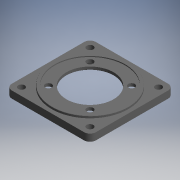
# Autodesk Inventor part: 2683767 EAMF-U-140A-120G-S1---(ADAX)
Saved by Autodesk Inventor 2017.3 (Build 213256000, 256)
## iProperties
Part Number: 2683767 EAMF-U-140A-120G-S1---(ADAX)
Material: Generic
Catalog Web Link: www.cadenas.de
Description: EAMF-U-E-xx-(ADAX)-adapter plate
Vendor: FESTO
Document SubType Name: Modeling
Designer: partserver
Manufacturer: FESTO
Mass: 144.189 g
Surface Area: 441.925 cm^2
Volume: 144.189 cm^3
Density: 1 g/cm^3
Appearance: PSOLRGB-128-128-128
Category: PARTsolutions
Company: FESTO
Title: 2683767 EAMF-U-140A-120G-S1---(ADAX)
Author: Cadenas PARTsolutions
Comments: adapter plate
PSOL_IDENT_0: {$CADENAS_DATA\23d-libs\festo\parts\e\eamm\parts\eamm_u_e_ad_ax.prj},225 {VTYP=3D},{NB=2683767 EAMF-
PSOL_IDENT_1: U-140A-120G-S1---(ADAX)},{LINA=2683767 EAMF-U-140A-120G-S1---(ADAX)},{NN=EAMF-U-E-xx-(ADAX)},{DATE=2
PSOL_IDENT_2: 6.02.2021 07:54:19},{GEOMDATE=26.02.2021 07:54:00},{VERSION=},{LINEID=160},{WBVAR=},{WBNUMERIC=}  {N
PSOL_IDENT_3: B=2683767 EAMF-U-140A-120G-S1---(ADAX)},{LINA=2683767 EAMF-U-140A-120G-S1---(ADAX)},{KT=DUMMY},{TNR=
PSOL_IDENT_4: 2683767},{TYP=EAMF-U-140A-120G-S1},{VERS=3},{B=15.500},{B1=3.500},{B2=9.000},{D1=100.000},{D2=165.00
PSOL_IDENT_5: 0},{D3=80.000},{D4=115.300},{D5=119.700},{D6=119.300},{D7=11.000},{D8=11.000},{D9=130.000},{E=143.00
PSOL_IDENT_6: 0},{W1=45.000},{H=0.000},{H1=0.000},{H2=0.000},{D10=0.000},{B3=0.000},{X1=0.000}
NB: 2683767 EAMF-U-140A-120G-S1---(ADAX)
NN: EAMF-U-E-xx-(ADAX)
NT: adapter plate
NBSYN: $TNR. $TYP.---(ADAX)
LINA: 2683767 EAMF-U-140A-120G-S1---(ADAX)
CATALOG: Festo
TNR: 2683767
TYP: EAMF-U-140A-120G-S1
D10: 0
B3: 0
X1: 0
SUPPLIER: FESTO
ARTICLENO: 2683767 EAMF-U-140A-120G-S1---(ADAX)
BOMINFO: 2683767 EAMF-U-140A-120G-S1---(ADAX)
CREATOR: CADENAS GmbH
Autodesk Inventor part; units mm, degrees
sketch "Sketch_1" plane through (0, 0, 0) normal (0, 0, 1) x (1, 0, 0)
  arc A0 (-71.5, -61.5) -> (-61.5, -71.5) centre (-61.5, -61.5) ccw
  line L0 (-61.5, -71.5) -> (61.5, -71.5)
  arc A1 (61.5, -71.5) -> (71.5, -61.5) centre (61.5, -61.5) ccw
  line L1 (71.5, -61.5) -> (71.5, 61.5)
  arc A2 (71.5, 61.5) -> (61.5, 71.5) centre (61.5, 61.5) ccw
  line L2 (61.5, 71.5) -> (-61.5, 71.5)
  arc A3 (-61.5, 71.5) -> (-71.5, 61.5) centre (-61.5, 61.5) ccw
  line L3 (-71.5, 61.5) -> (-71.5, -61.5)
  circle A4 centre (58.3363, 58.3363) radius 5.5
  circle A5 centre (58.3363, -58.3363) radius 5.5
  circle A6 centre (-58.3363, 58.3363) radius 5.5
  circle A7 centre (-58.3363, -58.3363) radius 5.5
  constraints: 8 centre point, 8 end point, 8 point on circle
extrude "Extrusion1" add sketch "Sketch_1" along normal blind 12
sketch "Sketch_2" plane through (0, 0, 0) normal (1, 0, 0) x (0, 1, 0)
  line L0 (0, -3.5) -> (0, 0)
  line L1 (0, 0) -> (65, 0)
  line L2 (65, 0) -> (65, -3.067)
  line L3 (65, -3.067) -> (64.75, -3.5)
  line L4 (64.75, -3.5) -> (0, -3.5)
  line L5 (0, -3.5) -> (0, 0)
  constraints: 12 end point
revolve "Revolution1" add sketch "Sketch_2" angle 360 about axis through (0, 0, -3.5) along (0, 0, -1)
sketch "Sketch3" plane through (0, 0, -3.5) normal (0, 0, -1) x (-1, 0, 0)
  point P0 (-35.3553, 35.3553)
hole "Hole1" at (35.3553, 35.3553, -3.5) direction (0, 0, 1) diameter 11 depth 15.5
pattern_linear "Rectangular Pattern1" count 2 spacing 70.7107 along (-1, 0, 0) count 2 spacing 70.7107 along (0, -1, 0) of "Hole1"
sketch "Sketch_7" plane through (0, 0, 0) normal (1, 0, 0) x (0, 1, 0)
  line L0 (0, -3.5) -> (0, 12)
  line L1 (0, 12) -> (60.4387, 12)
  arc A0 (60.4387, 12) -> (60.0057, 11.75) centre (60.4387, 11.5) ccw
  line L2 (60.0057, 11.75) -> (59.784, 11.366)
  arc A1 (59.784, 11.366) -> (59.65, 10.866) centre (60.65, 10.866) ccw
  line L3 (59.65, 10.866) -> (59.65, 10.4362)
  arc A2 (59.65, 10.4362) -> (59.6833, 10.1802) centre (60.65, 10.4362) ccw
  arc A3 (59.6572, 7.525) -> (59.6833, 10.1802) centre (54.85, 8.9) ccw
  arc A4 (58.6958, 6.8) -> (59.6572, 7.525) centre (58.6958, 7.8) ccw
  line L4 (58.6958, 6.8) -> (58.15, 6.8)
  line L5 (58.15, 6.8) -> (57.65, 6.3)
  line L6 (57.65, 6.3) -> (57.65, 3)
  line L7 (57.65, 3) -> (40.5, 3)
  line L8 (40.5, 3) -> (40, 2.5)
  line L9 (40, 2.5) -> (40, -3.5)
  line L10 (40, -3.5) -> (0, -3.5)
  line L11 (0, -3.5) -> (0, 12)
  constraints: 24 end point, 10 point on circle, 5 centre point
revolve "Revolution2" cut sketch "Sketch_7" angle 360 about axis through (0, 0, -3.5) along (0, 0, -1)
sketch "Sketch_16" plane through (0, 0, 0) normal (1, 0, 0) x (0, 1, 0)
  line L0 (0, -2) -> (0, -3.5)
  line L1 (0, -3.5) -> (-60, -3.5)
  line L2 (-60, -3.5) -> (-60, -2)
  line L3 (-60, -2) -> (0, -2)
  line L4 (0, -2) -> (0, -3.5)
  constraints: 10 end point
revolve "Revolution3" cut sketch "Sketch_16" angle 360 about axis through (0, 0, -2) along (0, 0, 1)
ref_plane "ANBAU_XY" through (0, 0, 0) normal (0, 0, 1) x (1, 0, 0)
ref_plane "ANBAU_YZ" through (0, 0, 0) normal (1, 0, 0) x (0, 1, 0)
ref_plane "ANBAU_ZX" through (0, 0, 0) normal (0, 1, 0) x (0, 0, 1)
ref_plane "M_SCREWS_1_XY" through (-35.3553, -35.3553, -3.5) normal (0, 0, 1) x (1, 0, 0)
ref_plane "M_SCREWS_1_YZ" through (-35.3553, -35.3553, -3.5) normal (1, 0, 0) x (0, 1, 0)
ref_plane "M_SCREWS_1_ZX" through (-35.3553, -35.3553, -3.5) normal (0, 1, 0) x (0, 0, 1)
ref_plane "M_SCREWS_2_XY" through (35.3553, -35.3553, -3.5) normal (0, 0, 1) x (1, 0, 0)
ref_plane "M_SCREWS_2_YZ" through (35.3553, -35.3553, -3.5) normal (1, 0, 0) x (0, 1, 0)
ref_plane "M_SCREWS_2_ZX" through (35.3553, -35.3553, -3.5) normal (0, 1, 0) x (0, 0, 1)
ref_plane "M_SCREWS_3_XY" through (35.3553, 35.3553, -3.5) normal (0, 0, 1) x (1, 0, 0)
ref_plane "M_SCREWS_3_YZ" through (35.3553, 35.3553, -3.5) normal (1, 0, 0) x (0, 1, 0)
ref_plane "M_SCREWS_3_ZX" through (35.3553, 35.3553, -3.5) normal (0, 1, 0) x (0, 0, 1)
ref_plane "M_SCREWS_4_XY" through (-35.3553, 35.3553, -3.5) normal (0, 0, 1) x (1, 0, 0)
ref_plane "M_SCREWS_4_YZ" through (-35.3553, 35.3553, -3.5) normal (1, 0, 0) x (0, 1, 0)
ref_plane "M_SCREWS_4_ZX" through (-35.3553, 35.3553, -3.5) normal (0, 1, 0) x (0, 0, 1)
ref_plane "RS_1_XY" through (58.3363, 58.3363, 12) normal (0, 0, 1) x (1, 0, 0)
ref_plane "RS_1_YZ" through (58.3363, 58.3363, 12) normal (1, 0, 0) x (0, 1, 0)
ref_plane "RS_1_ZX" through (58.3363, 58.3363, 12) normal (0, 1, 0) x (0, 0, 1)
ref_plane "RS_2_XY" through (-58.3363, 58.3363, 12) normal (0, 0, 1) x (1, 0, 0)
ref_plane "RS_2_YZ" through (-58.3363, 58.3363, 12) normal (1, 0, 0) x (0, 1, 0)
ref_plane "RS_2_ZX" through (-58.3363, 58.3363, 12) normal (0, 1, 0) x (0, 0, 1)
ref_plane "RS_3_XY" through (-58.3363, -58.3363, 12) normal (0, 0, 1) x (1, 0, 0)
ref_plane "RS_3_YZ" through (-58.3363, -58.3363, 12) normal (1, 0, 0) x (0, 1, 0)
ref_plane "RS_3_ZX" through (-58.3363, -58.3363, 12) normal (0, 1, 0) x (0, 0, 1)
ref_plane "RS_4_XY" through (58.3363, -58.3363, 12) normal (0, 0, 1) x (1, 0, 0)
ref_plane "RS_4_YZ" through (58.3363, -58.3363, 12) normal (1, 0, 0) x (0, 1, 0)
ref_plane "RS_4_ZX" through (58.3363, -58.3363, 12) normal (0, 1, 0) x (0, 0, 1)
ref_plane "S2_1_XY" through (58.3363, 58.3363, 12) normal (0, 0, -1) x (1, 0, 0)
ref_plane "S2_1_YZ" through (58.3363, 58.3363, 12) normal (1, 0, 0) x (0, -1, 0)
ref_plane "S2_1_ZX" through (58.3363, 58.3363, 12) normal (0, -1, 0) x (0, 0, -1)
ref_plane "S2_2_XY" through (-58.3363, 58.3363, 12) normal (0, 0, -1) x (1, 0, 0)
ref_plane "S2_2_YZ" through (-58.3363, 58.3363, 12) normal (1, 0, 0) x (0, -1, 0)
ref_plane "S2_2_ZX" through (-58.3363, 58.3363, 12) normal (0, -1, 0) x (0, 0, -1)
ref_plane "S2_3_XY" through (-58.3363, -58.3363, 12) normal (0, 0, -1) x (1, 0, 0)
ref_plane "S2_3_YZ" through (-58.3363, -58.3363, 12) normal (1, 0, 0) x (0, -1, 0)
ref_plane "S2_3_ZX" through (-58.3363, -58.3363, 12) normal (0, -1, 0) x (0, 0, -1)
ref_plane "S2_4_XY" through (58.3363, -58.3363, 12) normal (0, 0, -1) x (1, 0, 0)
ref_plane "S2_4_YZ" through (58.3363, -58.3363, 12) normal (1, 0, 0) x (0, -1, 0)
ref_plane "S2_4_ZX" through (58.3363, -58.3363, 12) normal (0, -1, 0) x (0, 0, -1)
body "Solid1"
